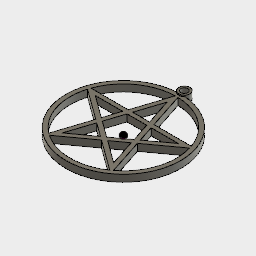
FPROJ_9_Czw (Autodesk Fusion 360 design; units mm, degrees)
Autodesk Fusion 360 part; units mm, degrees
sketch "草图1" plane through (0, 0, 0) normal (0, 1, 0) x (1, 0, 0)
sketch "草图2" plane through (0, 0, 0) normal (0, 1, 0) x (1, 0, 0)
  circle A0 centre (0, 0) radius 40.6099
  line L0 (0, 30.9017) -> (5.9631, 12.5492)
  line L1 (0.9789, 37.5972) -> (9.1175, 12.5492)
  line L2 (-0.9789, 37.5972) -> (-9.1175, 12.5492)
  line L3 (-10.0923, 9.5492) -> (-22.891, -29.8414)
  line L4 (0, 30.9017) -> (-5.9631, 12.5492)
  line L5 (-6.9379, 9.5492) -> (-18.1636, -25)
  line L6 (29.3893, 9.5492) -> (0, -11.8034)
  line L7 (-2.552, -13.6575) -> (-18.1636, -25)
  line L8 (36.0595, 10.6872) -> (2.552, -13.6575)
  line L9 (0, -15.5116) -> (-21.3071, -30.9921)
  line L10 (18.1636, -25) -> (-11.2257, -3.6475)
  line L11 (-13.7777, -1.7933) -> (-29.3893, 9.5492)
  line L12 (21.3071, -30.9921) -> (-12.2005, -6.6475)
  line L13 (-14.7524, -4.7933) -> (-36.0595, 10.6872)
  line L14 (6.9379, 9.5492) -> (11.2257, -3.6475)
  line L15 (12.2005, -6.6475) -> (18.1636, -25)
  line L16 (10.0923, 9.5492) -> (13.7777, -1.7933)
  line L17 (14.7524, -4.7933) -> (22.891, -29.8414)
  arc A1 (-36.0595, 10.6872) -> (-22.891, -29.8414) centre (0, 0) ccw
  arc A2 (-0.9789, 37.5972) -> (-35.4545, 12.5492) centre (0, 0) ccw
  arc A3 (-21.3071, -30.9921) -> (21.3071, -30.9921) centre (0, 0) ccw
  arc A4 (22.891, -29.8414) -> (36.0595, 10.6872) centre (0, 0) ccw
  arc A5 (35.4545, 12.5492) -> (0.9789, 37.5972) centre (0, 0) ccw
  line L18 (-35.4545, 12.5492) -> (5.9631, 12.5492)
  line L19 (9.1175, 12.5492) -> (35.4545, 12.5492)
  line L20 (-29.3893, 9.5492) -> (6.9379, 9.5492)
  line L21 (10.0923, 9.5492) -> (29.3893, 9.5492)
  point P0 (0, 30.9017)
  point P1 (-18.1636, -25)
  point P2 (-29.3893, 9.5492)
  point P3 (29.3893, 9.5492)
  point P4 (18.1636, -25)
sketch "草图3" plane through (0, 0, 0) normal (0, 1, 0) x (1, 0, 0)
extrude "拉伸1" add sketch "草图2" along normal blind 5 makes body 1
sketch "草图4" plane through (0, 0, 0) normal (0, 1, 0) x (1, 0, 0)
  circle A0 centre (65, 20) radius 2.5
  circle A1 centre (65, 20) radius 4
extrude "拉伸2" add sketch "草图4" along normal blind 5 separate body makes body 2
move_body "移动1" bodies 2 to x (1, 0, 0) y (0, 1, 0) z (0, 0, 1) at (-65.0082, 0.9152, -23.1466)
combine "合并1" operation add target body 2 tool bodies 1
